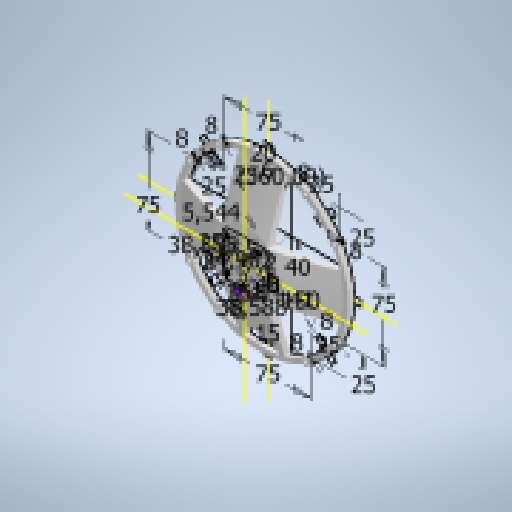
# Autodesk Inventor part: lidar_holder
Saved by Autodesk Inventor 2024.3 (Build 283343000, 343)
## iProperties
Created: 2026-05-03
Part Number: lidar_holder
Material: Generic
Document SubType Name: Modeling
Designer: owozn
Density: 1 g/cm^3
Appearance: Default
Author: owozn
Autodesk Inventor part; units mm, degrees
ref_plane "YZ Plane" through (0, 0, 0) normal (1, 0, 0) x (0, 1, 0)
ref_plane "XZ Plane" through (0, 0, 0) normal (0, 1, 0) x (-1, 0, 0)
ref_plane "XY Plane" through (0, 0, 0) normal (0, 0, 1) x (1, 0, 0)
sketch "Sketch1" plane through (0, 0, 0) normal (0, 0, 1) x (1, 0, 0)
  line L0 (-112.7, 0) -> (112.7, 0) projected
  line L1 (0, -112.7) -> (0, 112.7) projected
  circle A0 centre (0, 0) radius 70.5
  circle A1 centre (0, 0) radius 75
  line L2 (3, 80.5) -> (-3, 80.5)
  line L3 (-3, 80.5) -> (-3, 60.5)
  line L4 (-3, 60.5) -> (3, 60.5)
  line L5 (3, 60.5) -> (3, 80.5)
  line L6 (3, 80.5) -> (-3, 60.5) construction
  line L7 (-3, 80.5) -> (3, 60.5) construction
  line L8 (-40.6586, 44.9013) -> (-54.8008, 59.0434)
  line L9 (-54.8008, 59.0434) -> (-59.0434, 54.8008)
  line L10 (-59.0434, 54.8008) -> (-44.9013, 40.6586)
  line L11 (-59.0434, 54.8008) -> (-40.6586, 44.9013) construction
  line L12 (-54.8008, 59.0434) -> (-44.9013, 40.6586) construction
  line L13 (-44.9013, 40.6586) -> (-40.6586, 44.9013)
  line L14 (-60.5, 3) -> (-80.5, 3)
  line L15 (-80.5, 3) -> (-80.5, -3)
  line L16 (-80.5, -3) -> (-60.5, -3)
  line L17 (-80.5, -3) -> (-60.5, 3) construction
  line L18 (-80.5, 3) -> (-60.5, -3) construction
  line L19 (-60.5, -3) -> (-60.5, 3)
  line L20 (-44.9013, -40.6586) -> (-59.0434, -54.8008)
  line L21 (-59.0434, -54.8008) -> (-54.8008, -59.0434)
  line L22 (-54.8008, -59.0434) -> (-40.6586, -44.9013)
  line L23 (-54.8008, -59.0434) -> (-44.9013, -40.6586) construction
  line L24 (-59.0434, -54.8008) -> (-40.6586, -44.9013) construction
  line L25 (-40.6586, -44.9013) -> (-44.9013, -40.6586)
  line L26 (-3, -60.5) -> (-3, -80.5)
  line L27 (-3, -80.5) -> (3, -80.5)
  line L28 (3, -80.5) -> (3, -60.5)
  line L29 (3, -80.5) -> (-3, -60.5) construction
  line L30 (-3, -80.5) -> (3, -60.5) construction
  line L31 (3, -60.5) -> (-3, -60.5)
  line L32 (40.6586, -44.9013) -> (54.8008, -59.0434)
  line L33 (54.8008, -59.0434) -> (59.0434, -54.8008)
  line L34 (59.0434, -54.8008) -> (44.9013, -40.6586)
  line L35 (59.0434, -54.8008) -> (40.6586, -44.9013) construction
  line L36 (54.8008, -59.0434) -> (44.9013, -40.6586) construction
  line L37 (44.9013, -40.6586) -> (40.6586, -44.9013)
  line L38 (60.5, -3) -> (80.5, -3)
  line L39 (80.5, -3) -> (80.5, 3)
  line L40 (80.5, 3) -> (60.5, 3)
  line L41 (80.5, 3) -> (60.5, -3) construction
  line L42 (80.5, -3) -> (60.5, 3) construction
  line L43 (60.5, 3) -> (60.5, -3)
  line L44 (44.9013, 40.6586) -> (59.0434, 54.8008)
  line L45 (59.0434, 54.8008) -> (54.8008, 59.0434)
  line L46 (54.8008, 59.0434) -> (40.6586, 44.9013)
  line L47 (54.8008, 59.0434) -> (44.9013, 40.6586) construction
  line L48 (59.0434, 54.8008) -> (40.6586, 44.9013) construction
  line L49 (40.6586, 44.9013) -> (44.9013, 40.6586)
  line L50 (49.851, -49.851) -> (0, 0) construction
  circle A2 centre (-62.5, -37.5) radius 4
  circle A3 centre (-62.5, 37.5) radius 4
  circle A4 centre (-37.5, 62.5) radius 4
  circle A5 centre (37.5, 62.5) radius 4
  circle A6 centre (62.5, 37.5) radius 4
  circle A7 centre (62.5, -37.5) radius 4
  circle A8 centre (37.5, -62.5) radius 4
  circle A9 centre (-37.5, -62.5) radius 4
  line L51 (-20, 20) -> (20, 20)
  line L52 (20, 20) -> (20, -20)
  line L53 (20, -20) -> (-20, -20)
  line L54 (-20, -20) -> (-20, 20)
  line L55 (-20, 20) -> (20, -20) construction
  line L56 (20, 20) -> (-20, -20) construction
  line L57 (-20, 20) -> (-67.6036, 20)
  line L58 (-20, -20) -> (-67.6036, -20)
  line L59 (-20, -20) -> (-20, -67.6036)
  line L60 (20, -20) -> (20, -67.6036)
  line L61 (20, -20) -> (67.6036, -20)
  line L62 (20, 20) -> (67.6036, 20)
  line L63 (20, 20) -> (20, 67.6036)
  line L64 (-20, 20) -> (-20, 67.6036)
  arc A10 (14.9232, -68.984) -> (-14.9149, -68.9043) centre (0, -70.5) ccw
  point P0 (0, 0)
  point P1 (0, 70.5)
  point P2 (-49.851, 49.851)
  point P3 (-70.5, 0)
  point P4 (-49.851, -49.851)
  point P5 (49.851, -49.851)
  point P6 (70.5, 0)
  point P7 (49.851, 49.851)
  point P8 (35.593, -66.0162)
  point P9 (41.4999, -62.4721)
  point P10 (62.4721, -41.4999)
  point P11 (66.0162, -35.593)
  point P12 (66.0162, 35.593)
  point P13 (62.4721, 41.4999)
  point P14 (41.4999, 62.4721)
  point P15 (35.593, 66.0162)
  point P16 (-35.593, 66.0162)
  point P17 (-41.4999, 62.4721)
  point P18 (-62.4721, 41.4999)
  point P19 (-66.0162, 35.593)
  point P20 (-66.0162, -35.593)
  point P21 (-62.4721, -41.4999)
  point P22 (-41.4999, -62.4721)
  point P23 (-35.593, -66.0162)
  point P24 (-33.5293, -62.0164)
  point P25 (-38.9418, -58.7689)
  point P26 (-58.7689, -38.9418)
  point P27 (-62.0164, -33.5293)
  point P28 (-62.0164, 33.5293)
  point P29 (-58.7689, 38.9418)
  point P30 (-38.9418, 58.7689)
  point P31 (-33.5293, 62.0164)
  point P32 (33.5293, 62.0164)
  point P33 (38.9418, 58.7689)
  point P34 (58.7689, 38.9418)
  point P35 (62.0164, 33.5293)
  point P36 (62.0164, -33.5293)
  point P37 (58.7689, -38.9418)
  point P38 (38.9418, -58.7689)
  point P39 (33.5293, -62.0164)
  point P40 (0, 0)
  point P41 (14.9149, -68.9043)
  point P42 (3, 70.4361)
  point P43 (-3, 70.4361)
  point P44 (-70.4361, 3)
  point P45 (-70.4361, -3)
  point P46 (70.4361, -3)
  point P47 (70.4361, 3)
  point P48 (3, 74.94)
  point P49 (-3, 74.94)
  dimension "d2" = 141
  dimension "d3" = 150
  dimension "d4" = 6
  dimension "d5" = 20
  dimension "d6" = 360
  dimension "d7" = 25
  dimension "d8" = 25
  dimension "d9" = 75
  dimension "d10" = 25
  dimension "d11" = 25
  dimension "d12" = 25
  dimension "d13" = 25
  dimension "d14" = 75
  dimension "d15" = 25
  dimension "d16" = 25
  dimension "d17" = 75
  dimension "d18" = 75
  dimension "d19" = 8
  dimension "d20" = 8
  dimension "d21" = 8
  dimension "d22" = 8
  dimension "d23" = 8
  dimension "d24" = 8
  dimension "d25" = 8
  dimension "d26" = 8
  dimension "d36" = 40
  dimension "d37" = 40
  dimension "d45" = 15
  constraints: 126 end point, 12 coincident, 10 centre point, 7 parallel, 6 midpoint, 5 point on line, 3 horizontal, 3 perpendicular, 2 point on circle, 2 symmetric about line, 1 horizontal alignment, 101 other
  measures "d3" diameter of A1
  measures "d4" distance of L4.end L3.end
  measures "d5" distance of L3.end L2.end
  measures "d7" horizontal distance of point (62.5, -37.5) point (37.5, -62.5)
  measures "d8" horizontal distance of point (62.5, -37.5) point (37.5, -62.5)
  measures "d9" distance of point (-37.5, -62.5) point (37.5, -62.5)
  measures "d10" horizontal distance of point (-37.5, 62.5) point (-62.5, 37.5)
  measures "d11" horizontal distance of point (-37.5, 62.5) point (-62.5, 37.5)
  measures "d12" horizontal distance of point (62.5, 37.5) point (37.5, 62.5)
  measures "d13" horizontal distance of point (37.5, 62.5) point (62.5, 37.5)
  measures "d14" distance of point (62.5, 37.5) point (62.5, -37.5)
  measures "d15" horizontal distance of point (-62.5, -37.5) point (-37.5, -62.5)
  measures "d16" horizontal distance of point (-62.5, -37.5) point (-37.5, -62.5)
  measures "d17" distance of point (-62.5, -37.5) point (-62.5, 37.5)
  measures "d18" distance of point (37.5, 62.5) point (-37.5, 62.5)
  measures "d19" diameter of A2
  measures "d20" diameter of A3
  measures "d21" diameter of A4
  measures "d22" diameter of A5
  measures "d23" diameter of A6
  measures "d24" diameter of A7
  measures "d25" diameter of A8
  measures "d26" diameter of A9
  measures "d36" distance of L52.end L53.end
  measures "d37" distance of L51.end L52.end
  measures "d45" radius of A10
extrude "Extrusion1" add sketch "Sketch1" along normal blind 5 contours A0 L40 A1 L0 | L0 A1 L38 A0 | A0 A6 A1 L40 | L38 A1 A7 A0 | A6 A0 A1 | A1 A6 | A7 A1 | A1 A7 A0 | A6 A0 | A0 A7 | A6 A0 L44 A1 | A1 L34 A0 A7 | A0 L5 A1 A5 | A0 A8 A1 L28 | L44 A0 L46 A1 | A1 L32 A0 L34 | A5 A1 A0 | A0 A5 | A0 L1 A1 L5 | A8 A0 | A0 A8 A1 | L46 A0 A5 A1 | A1 A8 A0 L32 | A0 L16 A1 L0 | L0 A1 L14 A0 | A0 A2 A1 L16 | A0 L26 A1 A9 | A0 L14 A1 A3 | A0 A4 A1 L3 | A0 L3 A1 L1 | A5 A1 | L28 A1 L1 A0 | A1 A8 | A2 A0 | A0 A2 A1 | A9 A1 A0 | A0 A9 | A3 A1 A0 | A0 A3 | A4 A0 | A0 A4 A1 | L1 A1 L26 A0 | A0 L20 A1 A2 | A1 A2 | A9 A1 L22 A0 | A3 A1 L10 A0 | A3 A1 | A0 L8 A1 A4 | A0 L22 A1 L20 | A1 A9 | L10 A1 L8 A0 | A1 A4
hole "Hole1" at (-37.5, -62.5, 0) at (37.5, -62.5, 0) at (62.5, -37.5, 0) at (62.5, 37.5, 0) at (37.5, 62.5, 0) at (-37.5, 62.5, 0) at (-62.5, 37.5, 0) at (-62.5, -37.5, 0) direction (0, 0, 1) diameter 3.2 end through all
extrude "Extrusion2" add sketch "Sketch1" along normal blind 20 contours L52 L53 L1 L0 | L0 L1 L51 L52 | L1 L53 L54 L0 | L0 L54 L51 L1
extrude "Extrusion3" cut sketch "Sketch1" along normal blind 5 contours L52 L53 L1 L0 | L0 L1 L51 L52 | L1 L53 L54 L0 | L0 L54 L51 L1
sketch "Sketch2" plane through (-20, -20, 20) normal (-1, 0, 0) x (0, 0, 1)
  line L0 (-24, 20) -> (4, 20) projected
  line L1 (-20, -85) -> (-20, 125) projected
  line L2 (0, 22.5) -> (-5, 22.5)
  line L3 (-5, 22.5) -> (-5, 17.5)
  line L4 (-5, 17.5) -> (0, 17.5)
  line L5 (0, 17.5) -> (0, 22.5)
  line L6 (0, 22.5) -> (-5, 17.5) construction
  line L7 (-5, 22.5) -> (0, 17.5) construction
  point P0 (-20, 20)
  point P1 (-2.5, 20)
  dimension "d42" = 5
  dimension "d43" = 5
  dimension "d44" = 17.5
  constraints: 12 end point, 2 midpoint, 2 parallel, 1 horizontal, 1 perpendicular, 1 point on line
  measures "d42" distance of L4.end L3.end
  measures "d43" distance of L3.end L2.end
  measures "d44" distance from line of L1 point (-2.5, 20)
extrude "Extrusion4" add sketch "Sketch1" along normal blind 20 contours A0 L38 L43 L0 | L0 L43 L40 A0 | L43 L38 A0 L61 L52 L0 | L0 L52 L62 A0 L40 L43 | L51 L1 L4 L5 A0 L63 | L60 A0 A10 L1 L53 | L54 L58 A0 L16 L19 L0 | L0 L19 L14 A0 L57 L54 | L1 A10 A0 L59 L53 | L51 L64 A0 L3 L4 L1 | L19 L16 A0 L0 | L0 A0 L14 L19 | L4 L3 A0 L1 | L1 A0 L5 L4
chamfer "Chamfer1" distance 42 distance2 15 1 edges at (70.5, 0, 20) measured on face at (36.8333, 0, 20)
chamfer "Chamfer2" distance 42 distance2 15 1 edges at (-17.4695, -68.3013, 20) measured on face at (0, 36.8333, 20)
chamfer "Chamfer3" distance 42 distance2 15 1 edges at (-70.5, 0, 20) measured on face at (0, 36.8333, 20)
chamfer "Chamfer4" distance 42 distance2 15 1 edges at (0, 70.5, 20) measured on face at (0, 36.8333, 20)
sketch "Sketch3" plane through (0, 0, 0) normal (0, 1, 0) x (-1, 0, 0)
  line L0 (0, -4) -> (0, 24) projected
  line L1 (105, 0) -> (-105, 0) projected
  line L2 (20, 0) -> (70.5, 0)
  line L3 (0, 5) -> (0, 0)
  line L4 (0, 0) -> (20, 0)
  line L5 (70.5, 0) -> (25, 15)
  line L6 (25, 15) -> (0, 15)
  line L7 (0, 0) -> (0, 15)
  dimension "d60" = 70.5
  dimension "d62" = 15
  dimension "d63" = 25
  constraints: 12 end point, 3 collinear, 2 perpendicular, 2 point on line
  measures "d60" distance of L3.end L2.end
  measures "d62" distance from line of L3.end L6
  measures "d63" distance from line of L0 L5.end
revolve "Revolution1" cut sketch "Sketch3" angle 360 about axis through (0, 0, -10) along (0, 0, 1)
sketch "Sketch4" plane through (0, 0, 20) normal (0, 0, 1) x (1, 0, 0)
  line L0 (0, -105) -> (0, 105) projected
  line L1 (-105, 0) -> (105, 0) projected
  line L2 (13.75, 19.294) -> (-13.75, 19.294)
  line L3 (-19.294, 13.75) -> (-19.294, -13.75)
  line L4 (-13.75, -19.294) -> (13.75, -19.294)
  line L5 (19.294, -13.75) -> (19.294, 13.75)
  line L6 (19.294, 19.294) -> (-19.294, -19.294) construction
  line L7 (-19.294, 19.294) -> (19.294, -19.294) construction
  arc A0 (-13.75, 19.294) -> (-19.294, 13.75) centre (-13.75, 13.75) ccw
  arc A1 (19.294, 13.75) -> (13.75, 19.294) centre (13.75, 13.75) ccw
  arc A2 (13.75, -19.294) -> (19.294, -13.75) centre (13.75, -13.75) ccw
  arc A3 (-19.294, -13.75) -> (-13.75, -19.294) centre (-13.75, -13.75) ccw
  circle A4 centre (23.4, 0) radius 3.6
  circle A5 centre (-8.5, -23.4064) radius 3.6
  circle A6 centre (0, 0) radius 12.451 construction
  circle A7 centre (0, 0) radius 24.902
  circle A8 centre (-8.5, 23.4064) radius 3.6
  circle A9 centre (-23.4, 0) radius 3.6
  circle A10 centre (8.5, -23.4064) radius 3.6
  circle A11 centre (8.5, 23.4064) radius 3.6
  dimension "d71" = 49.804
  dimension "d64" = 38.588
  dimension "d65" = 38.588
  dimension "d66" = 5.544
  dimension "d67" = 7.2
  dimension "d68" = 23.4
  dimension "d69" = 7.2
  dimension "d70" = 24.902
  dimension "d72" = 8.5
  constraints: 12 end point, 11 centre point, 9 point on line, 8 point on circle, 8 tangent, 4 symmetric about line, 3 equal radius, 2 coincident, 2 midpoint, 2 parallel, 1 horizontal, 1 perpendicular, 7 other
  measures "d64" distance of L6.end L7.end
  measures "d65" distance of L7.start L6.end
  measures "d66" radius of A0
  measures "d67" diameter of A4
  measures "d68" distance of point (0, 0) A4.centre
  measures "d69" diameter of A5
  measures "d70" diameter of A6
  measures "d72" distance from line of L0 A5.centre
hole "Hole2" at (-8.5, 23.4064, 20) at (8.5, 23.4064, 20) at (23.4, 0, 20) at (8.5, -23.4064, 20) at (-8.5, -23.4064, 20) at (-23.4, 0, 20) direction (0, 0, -1) diameter 3.2 end through all
body "Solid1"
